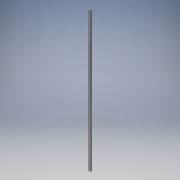
# Autodesk Inventor part: Track
Saved by Autodesk Inventor 2016 (Build 200138000, 138)
## iProperties
Created: 2016-10-31
Part Number: Track
Material: Generic
Document SubType Name: Modeling
Designer: mattc
Density: 1 g/cm^3
Appearance: Aluminum - Polished
Author: mattc
Autodesk Inventor part; units mm, degrees
ref_plane "YZ Plane" through (0, 0, 0) normal (1, 0, 0) x (0, 1, 0)
ref_plane "XZ Plane" through (0, 0, 0) normal (0, 1, 0) x (-1, 0, 0)
ref_plane "XY Plane" through (0, 0, 0) normal (0, 0, 1) x (1, 0, 0)
sketch "Sketch1" plane through (0, 0, 0) normal (0, 0, 1) x (1, 0, 0)
  line L0 (-9.49, 0.83) -> (9.49, 0.83)
  line L1 (11.15, 1.3646) -> (11.15, -0.83)
  line L2 (11.15, -0.83) -> (-11.15, -0.83)
  line L3 (-11.15, -0.83) -> (-11.15, 1.0973)
  line L4 (-9.49, 0.83) -> (-9.49, 13.67)
  line L5 (-9.49, 13.67) -> (-11.15, 13.67)
  line L6 (-11.15, 13.67) -> (-11.15, 1.0973)
  line L7 (9.49, 0.83) -> (9.49, 13.67)
  line L8 (9.49, 13.67) -> (11.15, 13.67)
  line L9 (11.15, 13.67) -> (11.15, 1.3646)
  point P0 (0, 0)
  point P1 (0, 0)
  dimension "d0" = 22.3
  dimension "d1" = 11.15
  dimension "d3" = 0.83
  dimension "d4" = 14.5
  dimension "d5" = 1.66
  dimension "d6" = 1.66
  dimension "d7" = 14.5
  dimension "d10" = 1.66
  constraints: 20 end point, 5 perpendicular, 4 parallel, 1 coincident, 1 horizontal
  measures "d0" distance of L1.end L2.end
  measures "d1" distance from line of L3 point (0, 0)
  measures "d3" distance from line of L2 point (0, 0)
  measures "d4" distance of L5.end L2.end
  measures "d5" distance of L4.end L5.end
  measures "d6" distance of L7.end L8.end
  measures "d7" distance of L1.end L8.end
  measures "d10" distance between parallel lines of L2 L0
extrude "Extrusion1" add sketch "Sketch1" along normal mid plane 1220
equation "\"d1\" = 0.5 * d0"
equation "\"d3\" = 0.5 * d10"
equation "\"d6\" = d5"
equation "\"d7\" = d4"
equation "\"d10\" = d5"
body "Solid1"
